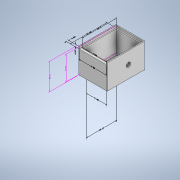
# Autodesk Inventor part: Part1
Saved by Autodesk Inventor 2022.6 (Build 266554010, 554A)
## iProperties
Created: 2025-05-13
Part Number: Part1
Material: Generic
Document SubType Name: Modeling
Designer: khinm
Density: 1 g/cm^3
Appearance: Default
Author: khinm
Autodesk Inventor part; units mm, degrees
ref_plane "XZ Plane" through (0, 0, 0) normal (0, 1, 0) x (-1, 0, 0)
sketch "Sketch1" plane through (0, 0, 0) normal (0, 0, 1) x (1, 0, 0)
  line L0 (-41, 37.5) -> (41, 37.5)
  line L1 (41, 37.5) -> (41, -37.5)
  line L2 (41, -37.5) -> (-41, -37.5)
  line L3 (-41, -37.5) -> (-41, 37.5)
  point P0 (0, 0)
  point P1 (0, 37.5)
  point P2 (-41, 0)
  dimension "d0" = 82
  dimension "d1" = 75
  constraints: 8 end point, 2 midpoint, 2 parallel, 1 horizontal, 1 horizontal alignment, 1 perpendicular, 1 vertical alignment
  measures "d0" distance of L0.start L0.end
  measures "d1" distance of L0.end L1.end
extrude "Extrusion1" add sketch "Sketch1" along normal mid plane 107
sketch "Sketch2" plane through (-41, 37.5, 53.5) normal (0, 1, 0) x (1, 0, 0)
  line L0 (0, 107) -> (82, 107) projected
  line L1 (6, 101) -> (76, 101)
  line L2 (76, 101) -> (76, 6)
  line L3 (76, 6) -> (6, 6)
  line L4 (6, 6) -> (6, 101)
  line L5 (0, 107) -> (0, 0) projected
  point P0 (41, 53.5)
  point P1 (41, 101)
  point P2 (41, 107)
  point P3 (6, 53.5)
  point P4 (0, 53.5)
  dimension "d4" = 95
  dimension "d5" = 70
  constraints: 8 end point, 4 midpoint, 2 parallel, 1 horizontal, 1 horizontal alignment, 1 perpendicular, 1 vertical alignment
  measures "d4" distance of L1.end L2.end
  measures "d5" distance of L1.start L1.end
extrude "Extrusion2" cut sketch "Sketch2" against normal blind 68
sketch "Sketch3" plane through (0, 0, 53.5) normal (0, 0, 1) x (1, 0, 0)
  line L0 (-35, 37.5) -> (35, 37.5)
  line L1 (35, 37.5) -> (35, 28.5)
  line L2 (35, 28.5) -> (-35, 28.5)
  line L3 (-35, 28.5) -> (-35, 37.5)
  line L4 (41, 37.5) -> (-41, 37.5) projected
  point P0 (0, 0)
  point P1 (0, 37.5)
  dimension "d14" = 70
  dimension "d15" = 9
  constraints: 8 end point, 2 midpoint, 2 parallel, 1 horizontal, 1 perpendicular
  measures "d14" distance of L1.end L2.end
  measures "d15" distance of L0.end L1.end
extrude "Extrusion3" cut sketch "Sketch3" against normal up to surface (6 mm away)
ref_plane "Work Plane1" through (0, 0, 0) normal (0, 0, 1) x (1, 0, 0)
sketch "Sketch5" plane through (0, 0, 0) normal (0, 0, 1) x (1, 0, 0)
  line L0 (-35, 37.5) -> (-35, -30.5) projected
  line L1 (-38, 34.5) -> (-35, 34.5)
  line L2 (-35, 34.5) -> (-35, 28.5)
  line L3 (-35, 28.5) -> (-38, 28.5)
  line L4 (-38, 28.5) -> (-38, 34.5)
  point P0 (0, 0)
  dimension "d21" = 3
  dimension "d22" = 6
  dimension "d23" = 3
  constraints: 8 end point, 2 parallel, 1 horizontal, 1 perpendicular, 1 point on line
  measures "d21" distance of L0.start L1.end
  measures "d22" distance of L1.start L3.end
  measures "d23" distance of L2.end L3.end
sketch3d "3D Sketch1"
  line L0 (-35, 37.5, 53.5) -> (-35, 37.5, -47.5)
  line L1 (-35, 37.5, -47.5) -> (35, 37.5, -47.5)
  line L2 (35, 37.5, -47.5) -> (35, 37.5, 53.5)
sweep "Sweep1" cut profiles "Sketch5" path "3D Sketch1"
ref_plane "Work Plane2" through (0, 0, 0) normal (1, 0, 0) x (0, 1, 0)
fillet "Fillet1" radius 2 10 edges at (41, 37.5, 0) (0, 37.5, -53.5) (-41, 37.5, 0) (41, 0, -53.5) (41, 0, 53.5) (-41, 0, 53.5) (-41, 0, -53.5) (35, 37.5, 3) (0, 37.5, -47.5) (-35, 37.5, 3)
fillet "Fillet2" radius 2 8 edges at (40.4142, -37.5, 52.9142) (0, -37.5, 53.5) (-40.4142, -37.5, 52.9142) (-41, -37.5, 0) (-40.4142, -37.5, -52.9142) (0, -37.5, -53.5) (40.4142, -37.5, -52.9142) (41, -37.5, 0)
sketch "Sketch9" plane through (-41, -30.5, 53.5) normal (0, 1, 0) x (1, 0, 0)
  line L0 (10.5, 98.5) -> (71.5, 98.5)
  line L1 (71.5, 98.5) -> (71.5, 8.5)
  line L2 (71.5, 8.5) -> (10.5, 8.5)
  line L3 (10.5, 8.5) -> (10.5, 98.5)
  point P0 (41, 53.5)
  point P1 (41, 96.5)
  point P2 (12.5, 53.5)
  point P3 (10.5, 53.5)
  point P4 (41, 98.5)
  dimension "d48" = 90
  dimension "d49" = 61
  constraints: 8 end point, 2 horizontal alignment, 2 midpoint, 2 parallel, 2 vertical alignment, 1 horizontal, 1 perpendicular
  measures "d48" distance of L0.end L1.end
  measures "d49" distance of L1.end L2.end
extrude "Extrusion5" add sketch "Sketch9" along normal blind 2.5
sketch "Sketch10" plane through (-41, -28, 53.5) normal (0, 1, 0) x (1, 0, 0)
  line L0 (71.5, 98.5) -> (10.5, 98.5) projected
  line L1 (12.5, 96.5) -> (69.5, 96.5)
  line L2 (69.5, 96.5) -> (69.5, 10.5)
  line L3 (69.5, 10.5) -> (12.5, 10.5)
  line L4 (12.5, 10.5) -> (12.5, 96.5)
  point P0 (41, 53.5)
  point P1 (12.5, 53.5)
  point P2 (41, 96.5)
  dimension "d52" = 57
  dimension "d53" = 86
  constraints: 8 end point, 2 midpoint, 2 parallel, 1 horizontal, 1 horizontal alignment, 1 perpendicular, 1 vertical alignment
  measures "d52" distance of L1.start L1.end
  measures "d53" distance of L1.end L2.end
extrude "Extrusion6" cut sketch "Sketch10" against normal up to surface (2.5 mm away)
fillet "Fillet3" radius 1 8 edges at (0, -28, -45) (0, -28, -43) (-30.5, -28, 0) (-28.5, -28, 0) (0, -28, 43) (0, -28, 45) (28.5, -28, 0) (30.5, -28, 0)
sketch "Sketch12" plane through (35, -30.5, -47.5) normal (-1, 0, 0) x (0, 0, 1)
  circle A0 centre (41, 30) radius 5.25
  line L0 (4.5, 1.5) -> (4.5, 0) projected
  line L1 (90.5, 0) -> (4.5, 0) projected
  point P0 (47.5, 30.5)
  dimension "d64" = 36.5
  dimension "d65" = 10.5
  dimension "d66" = 30
  constraints: 1 centre point
  measures "d64" distance from line of L0 A0.centre
  measures "d65" diameter of A0
  measures "d66" distance from line of L1 A0.centre
extrude "Extrusion7" cut sketch "Sketch12" against normal up to surface (6 mm away)
chamfer "Chamfer1" distance 1 angle 45 1 edges at (41, -0.5, -11.75)
chamfer "Chamfer2" distance 1 angle 45 1 edges at (35, -0.5, -11.75)
body "Solid1"
